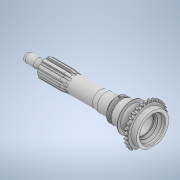
# Autodesk Inventor part: 68. Первичный вал
Saved by Autodesk Inventor 2021 (Build 250183000, 183)
## iProperties
Created: 2021-03-21
Part Number: 68. Первичный вал
Material: Типовые
Document SubType Name: Modeling
Designer: Данил
Density: 1 g/cm^3
Appearance: По умолчанию
Author: Данил
Autodesk Inventor part; units mm, degrees
sketch "Эскиз1" plane through (0, 0, 0) normal (0, 0, 1) x (1, 0, 0)
  line L0 (-123.25, 0) -> (123.25, 0)
  line L1 (-123.25, 0) -> (-123.25, -7.4282)
  line L2 (-119.25, -8.5) -> (-102.35, -8.5)
  line L3 (-119.25, -8.5) -> (-123.25, -7.4282)
  line L4 (-102.25, -8.6) -> (-102.25, -8.65)
  line L5 (-102.15, -8.75) -> (-91.25, -8.75)
  arc A0 (-102.25, -8.6) -> (-102.35, -8.5) centre (-102.35, -8.6) ccw
  arc A1 (-102.25, -8.65) -> (-102.15, -8.75) centre (-102.15, -8.65) ccw
  line L6 (-89.25, -10.75) -> (-89.25, -17.5)
  line L7 (-89.25, -17.5) -> (-43.25, -17.5)
  arc A2 (-89.25, -10.75) -> (-91.25, -8.75) centre (-91.25, -10.75) ccw
  line L8 (-43.25, -17.5) -> (-32.5769, -16)
  line L9 (-32.5769, -16) -> (20.5769, -16)
  line L10 (20.5769, -16) -> (31.25, -17.5)
  line L11 (31.25, -17.5) -> (50.5, -17.5)
  line L12 (50.5, -17.5) -> (50.6036, -17.3964)
  line L13 (50.9571, -17.25) -> (52.75, -17.25)
  line L14 (53.75, -18.25) -> (53.75, -21.5)
  arc A3 (50.9571, -17.25) -> (50.6036, -17.3964) centre (50.9571, -17.75) ccw
  arc A4 (53.75, -18.25) -> (52.75, -17.25) centre (52.75, -18.25) ccw
  line L15 (54.75, -22.5) -> (60.75, -22.5)
  line L16 (54.75, -22.5) -> (53.75, -21.5)
  line L17 (60.75, -22.5) -> (61.7036, -21.5464)
  line L18 (62.0571, -21.4) -> (63.35, -21.4)
  line L19 (64.35, -22.4) -> (64.35, -22.5)
  arc A5 (62.0571, -21.4) -> (61.7036, -21.5464) centre (62.0571, -21.9) ccw
  arc A6 (64.35, -22.4) -> (63.35, -21.4) centre (63.35, -22.4) ccw
  line L20 (64.35, -22.5) -> (78.1, -22.5)
  line L21 (78.1, -22.5) -> (78.2036, -22.3964)
  line L22 (78.5571, -22.25) -> (80.35, -22.25)
  line L23 (81.35, -23.25) -> (81.35, -28.25)
  arc A7 (78.5571, -22.25) -> (78.2036, -22.3964) centre (78.5571, -22.75) ccw
  arc A8 (81.35, -23.25) -> (80.35, -22.25) centre (80.35, -23.25) ccw
  line L24 (81.35, -28.25) -> (82.45, -28.25)
  line L25 (82.45, -28.25) -> (82.45, -36.4175)
  line L26 (82.45, -36.4175) -> (102.35, -36.4175)
  line L27 (102.35, -36.4175) -> (102.35, -30)
  line L28 (104.35, -28) -> (104.85, -28)
  line L29 (106.85, -30) -> (106.85, -40.5)
  arc A9 (104.35, -28) -> (102.35, -30) centre (104.35, -30) ccw
  arc A10 (106.85, -30) -> (104.85, -28) centre (104.85, -30) ccw
  line L30 (106.85, -40.5) -> (112.35, -40.5)
  line L31 (112.35, -40.5) -> (112.35, -32)
  line L32 (112.35, -32) -> (123.25, -31.5)
  line L33 (123.25, -31.5) -> (123.25, -26)
  line L34 (123.25, -26) -> (121.5179, -25)
  line L35 (121.5179, -25) -> (116.25, -25)
  line L36 (112.25, -21) -> (112.25, -20.4047)
  arc A11 (112.25, -21) -> (116.25, -25) centre (116.25, -21) ccw
  line L37 (112.25, -20.4047) -> (110.25, -19.25)
  line L38 (110.25, -19.25) -> (107.85, -19.25)
  line L39 (105.05, -19.25) -> (88.95, -19.25)
  line L40 (88.95, -19.25) -> (88.95, -19.75)
  line L41 (88.95, -19.75) -> (86.45, -19.75)
  line L42 (86.45, -19.75) -> (86.45, -15.6547)
  line L43 (86.45, -15.6547) -> (84.45, -14.5)
  line L44 (84.45, -14.5) -> (79.25, -14.5)
  line L45 (79.25, -14.5) -> (70.8784, 0)
  line L46 (105.05, -19.25) -> (105.05, -20.75)
  line L47 (106.05, -21.75) -> (106.85, -21.75)
  line L48 (107.85, -20.75) -> (107.85, -19.25)
  arc A12 (105.05, -20.75) -> (106.05, -21.75) centre (106.05, -20.75) ccw
  arc A13 (106.85, -21.75) -> (107.85, -20.75) centre (106.85, -20.75) ccw
  point P0 (0, 0)
  point P1 (0, 0)
  point P2 (-123.25, -8.5)
  point P3 (50.75, -17.25)
  point P4 (53.75, -22.5)
  point P5 (61.85, -21.4)
  point P6 (78.35, -22.25)
  point P7 (106.45, -21.75)
  dimension "d0" = 246.5
  dimension "d1" = 17
  dimension "d2" = 4
  dimension "d3" = 15
  dimension "d4" = 17.5
  dimension "d5" = 21
  dimension "d6" = 0.1
  dimension "d7" = 35
  dimension "d8" = 2
  dimension "d9" = 46
  dimension "d10" = 8
  dimension "d11" = 32
  dimension "d12" = 8
  dimension "d13" = 35
  dimension "d14" = 34
  dimension "d15" = 45
  dimension "d16" = 3
  dimension "d17" = 34.5
  dimension "d18" = 0.5
  dimension "d19" = 1
  dimension "d20" = 69.5
  dimension "d21" = 1
  dimension "d22" = 45
  dimension "d23" = 45
  dimension "d24" = 7
  dimension "d25" = 45
  dimension "d26" = 2.5
  dimension "d27" = 0.5
  dimension "d28" = 1
  dimension "d29" = 42.8
  dimension "d30" = 45
  dimension "d31" = 45
  dimension "d32" = 3
  dimension "d33" = 0.5
  dimension "d34" = 1
  dimension "d35" = 44.5
  dimension "d36" = 17
  dimension "d37" = 56.5
  dimension "d38" = 1.1
  dimension "d39" = 72.835
  dimension "d40" = 2
  dimension "d41" = 2
  dimension "d42" = 81
  dimension "d43" = 5.5
  dimension "d44" = 64
  dimension "d45" = 56
  dimension "d46" = 63
  dimension "d47" = 21
  dimension "d48" = 31
  dimension "d50" = 52
  dimension "d51" = 50
  dimension "d52" = 30
  dimension "d53" = 11
  dimension "d54" = 4
  dimension "d55" = 38.5
  dimension "d56" = 30
  dimension "d57" = 2
  dimension "d59" = 2.8
  dimension "d60" = 39.5
  dimension "d61" = 2.5
  dimension "d63" = 30
  dimension "d64" = 2
  dimension "d65" = 60
  dimension "d66" = 29
  constraints: 98 end point, 28 point on circle, 28 tangent, 15 horizontal, 14 centre point, 13 perpendicular, 11 point on line, 8 vertical, 2 coincident, 2 equal radius, 2 midpoint, 1 horizontal alignment, 1 vertical alignment
  measures "d0" distance of L0.start L0.end
  measures "d1" diameter of L2 L0
  measures "d2" distance of L2.start point (-123.25, -8.5)
  measures "d3" angle of L2 L3
  measures "d4" diameter of L5 L0
  measures "d5" distance from line of L0.start L4
  measures "d6" radius of A0
  measures "d7" diameter of L7 L0
  measures "d8" radius of A2
  measures "d9" distance from line of L7.end L6
  measures "d10" angle of L9 L8
  measures "d11" diameter of L9 L0
  measures "d12" angle of L11 L10
  measures "d13" diameter of L11 L0
  measures "d14" distance from line of L0.start L6
  measures "d15" angle of L14 L12
  measures "d16" distance from line of L14 point (50.75, -17.25)
  measures "d17" diameter of L13 L0
  measures "d18" radius of A3
  measures "d19" radius of A4
  measures "d20" distance from line of L0.end L14
  measures "d21" distance of L15.start point (53.75, -22.5)
  measures "d22" angle of L15 L16
  measures "d23" diameter of L15 L0
  measures "d24" distance from line of L15.end L14
  measures "d25" angle of L19 L17
  measures "d26" distance from line of L19 point (61.85, -21.4)
  measures "d27" radius of A5
  measures "d28" radius of A6
  measures "d29" diameter of L18 L0
  measures "d30" diameter of L20 L0
  measures "d31" angle of L21 L23
  measures "d32" distance from line of L23 point (78.35, -22.25)
  measures "d33" radius of A7
  measures "d34" radius of A8
  measures "d35" diameter of L22 L0
  measures "d36" distance between parallel lines of L23 L19
  measures "d37" diameter of L24 L0
  measures "d38" distance of L23.end L24.end
  measures "d39" diameter of L26 L0
  measures "d40" radius of A9
  measures "d41" radius of A10
  measures "d42" diameter of L30 L0
  measures "d43" distance of L29.end L30.end
  measures "d44" diameter of L31.end L0
  measures "d45" diameter of L28 L0
  measures "d46" diameter of L32.end L0
  measures "d47" distance between parallel lines of L27 L23
  measures "d48" distance between parallel lines of L31 L23
  measures "d50" diameter of L33.end L0
  measures "d51" diameter of L34.end L0
  measures "d52" angle of L35 L34
  measures "d53" distance between parallel lines of L36 L33
  measures "d54" radius of A11
  measures "d55" diameter of L38 L0
  measures "d56" angle of L38 L37
  measures "d57" horizontal distance of L36.end L37.end
  measures "d59" distance of L38.end L39.start
  measures "d60" diameter of L41 L0
  measures "d61" distance of L40.end L41.end
  measures "d63" angle of L39 L43
  measures "d64" distance from line of L43.end L42
  measures "d65" angle of L0 L45
  measures "d66" diameter of L44 L0
revolve "Вращение1" add sketch "Эскиз1" angle 360 about axis through (-123.25, 0, 0) along (1, 0, 0)
thread "Резьба1" size "M45x1.5" class "6g" standard "ISO Metric profile" full length
ref_plane "РабПлоскость1" through (104.6, 0, 0) normal (-1, 0, 0) x (0, 0, 1)
sketch "Эскиз2" plane through (104.6, 0, 0) normal (-1, 0, 0) x (0, 0, 1)
  line L0 (8, 36.4175) -> (-8, 36.4175) construction
  circle A0 centre (0, 0) radius 36.4175 projected
  line L1 (8, -35.5279) -> (8, 35.5279)
  line L2 (-8, 35.5279) -> (-8, -35.5279)
  line L3 (-8, 26.8328) -> (-9.5, 26.8328)
  line L4 (-9.5, 26.8328) -> (-9.5, 16.7425)
  line L5 (-9.5, 16.7425) -> (-8, 16.7425)
  circle A1 centre (0, 0) radius 28 projected
  circle A2 centre (0, 0) radius 19.25 projected
  line L6 (8, -16.6854) -> (9.6, -16.6854)
  line L7 (9.6, -16.6854) -> (9.6, -26.8328)
  line L8 (9.6, -26.8328) -> (8, -26.8328)
  point P0 (0, 36.4175)
  dimension "d74" = 16
  dimension "d75" = 3
  dimension "d76" = 3.2
  constraints: 18 end point, 8 point on circle, 4 horizontal, 4 point on line, 3 perpendicular, 3 vertical alignment, 2 vertical, 1 midpoint, 1 tangent
  measures "d74" distance of L0.start L0.end
  measures "d75" diameter of L4 L2
  measures "d76" diameter of L7 L1
revolve "Вращение2" cut sketch "Эскиз2" angle 360 about axis through (104.6, -35.5279, 8) along (0, 1, 0) picked at (8.7139, -20.3543) picked at (8.8918, -16.7824) contours L1 A2 L7 A1 | A1 L7 L8 | L1 L6 A2
revolve "Вращение3" cut sketch "Эскиз2" angle 360 about axis through (104.6, 35.5279, -8) along (0, -1, 0) picked at (-8.6691, 20.372) picked at (-8.8359, 16.8325) contours A1 L4 L3 | L2 A2 L4 A1 | L2 L5 A2
sketch "Эскиз3" plane through (0, 0, 0) normal (0, 0, 1) x (1, 0, 0)
  line L0 (50.5, 17.5) -> (31.25, 17.5) projected
  line L1 (70.8784, 0) -> (79.25, -14.5) projected
  line L2 (83.9986, -8.3348) -> (48.5273, 22.5)
  line L3 (70.8784, 0) -> (79.25, 14.5) projected
  line L4 (64.3813, 5.6018) -> (64.3663, 5.5844)
  line L5 (64.3311, 5.5818) -> (46.8871, 20.6132)
  line L6 (60.75, 22.5) -> (54.75, 22.5) projected
  line L7 (46.8871, 20.6132) -> (48.5273, 22.5)
  line L8 (78.1, -22.5) -> (64.35, -22.5) projected
  arc A0 (64.3311, 5.5818) -> (64.3663, 5.5844) centre (64.3474, 5.6007) ccw
  arc A1 (64.4166, 5.6044) -> (64.3813, 5.6018) centre (64.4003, 5.5855) ccw
  line L9 (83.9986, -8.3348) -> (82.4916, -10.0723)
  line L10 (64.4166, 5.6044) -> (82.4916, -10.0723)
  point P0 (0, 0)
  point P1 (64.35, 5.5655)
  point P2 (72.0587, 2.0444)
  point P3 (64.3659, 5.584)
  dimension "d79" = 41
  dimension "d81" = 4.8
  dimension "d82" = 5
  dimension "d83" = 0.025
  dimension "d89" = 4.6
  dimension "d90" = 47
  constraints: 12 end point, 4 point on circle, 4 point on line, 4 tangent, 3 perpendicular, 2 centre point, 1 equal radius, 1 horizontal alignment, 1 vertical alignment
  measures "d79" angle of L0 L2
  measures "d81" diameter of point (64.35, 5.565) L2
  measures "d82" diameter of L5.end L2
  measures "d83" radius of A0
  measures "d89" diameter of L9.end L2
  measures "d90" distance of L2.start L2.end
revolve "Вращение4" cut sketch "Эскиз3" angle 360 about axis through (83.9986, -8.3348, 0) along (-0.7547096, 0.656059, 0)
sketch "Эскиз4" plane through (0, 0, 0) normal (0, 0, 1) x (1, 0, 0)
  line L0 (60.75, 22.5) -> (54.75, 22.5) projected
  line L1 (53.75, 18.0823) -> (53.75, -18.25) projected
  line L2 (53.75, 18.0823) -> (53.75, 21.2451) projected
  arc A0 (53.75, 19.5) -> (60.75, 22.5) centre (41.5648, 57.5988) ccw
  line L3 (54.75, 22.5) -> (53.75, 21.5) projected
  line L4 (53.75, 21.5) -> (53.75, -21.5) projected
  point P0 (0, 0)
  dimension "d85" = 40
  dimension "d86" = 3
  constraints: 2 point on circle, 1 centre point, 1 point on line
  measures "d85" radius of A0
  measures "d86" vertical distance of L0.start A0.start
extrude "Выдавливание1" cut sketch "Эскиз4" along normal mid plane 3
sketch "Эскиз5" plane through (-89.25, 0, 0) normal (-1, 0, 0) x (0, 0, 1)
  circle A0 centre (0, 0) radius 17.5 projected
  circle A1 centre (0, 0) radius 13.25
  line L0 (-1.4483, 13.1706) -> (-2.7827, 17.2773)
  line L1 (-6.5698, 11.5065) -> (-7.9041, 15.6133)
  line L2 (-6.5698, 11.5065) -> (-1.4483, 13.1706) construction
  line L3 (-8.9132, 9.8039) -> (-12.4066, 12.342)
  line L4 (-12.0784, 5.4474) -> (-15.5718, 7.9855)
  line L5 (-12.0784, 5.4474) -> (-8.9132, 9.8039) construction
  line L6 (-12.9735, 2.6925) -> (-17.2916, 2.6925)
  line L7 (-12.9735, -2.6925) -> (-17.2916, -2.6925)
  line L8 (-12.9735, -2.6925) -> (-12.9735, 2.6925) construction
  line L9 (-12.0784, -5.4474) -> (-15.5718, -7.9855)
  line L10 (-8.9132, -9.8039) -> (-12.4066, -12.342)
  line L11 (-8.9132, -9.8039) -> (-12.0784, -5.4474) construction
  line L12 (-6.5698, -11.5065) -> (-7.9041, -15.6133)
  line L13 (-1.4483, -13.1706) -> (-2.7827, -17.2773)
  line L14 (-1.4483, -13.1706) -> (-6.5698, -11.5065) construction
  line L15 (1.4483, -13.1706) -> (2.7827, -17.2773)
  line L16 (6.5698, -11.5065) -> (7.9041, -15.6133)
  line L17 (6.5698, -11.5065) -> (1.4483, -13.1706) construction
  line L18 (8.9132, -9.8039) -> (12.4066, -12.342)
  line L19 (12.0784, -5.4474) -> (15.5718, -7.9855)
  line L20 (12.0784, -5.4474) -> (8.9132, -9.8039) construction
  line L21 (12.9735, -2.6925) -> (17.2916, -2.6925)
  line L22 (12.9735, 2.6925) -> (17.2916, 2.6925)
  line L23 (12.9735, 2.6925) -> (12.9735, -2.6925) construction
  line L24 (12.0784, 5.4474) -> (15.5718, 7.9855)
  line L25 (8.9132, 9.8039) -> (12.4066, 12.342)
  line L26 (8.9132, 9.8039) -> (12.0784, 5.4474) construction
  line L27 (6.5698, 11.5065) -> (7.9041, 15.6133)
  line L28 (1.4483, 13.1706) -> (2.7827, 17.2773)
  line L29 (1.4483, 13.1706) -> (6.5698, 11.5065) construction
  line L30 (-1.4483, 13.1706) -> (1.4483, 13.1706) construction
  point P0 (0, 13.1706)
  dimension "d92" = 26.5
  dimension "d93" = 5.385
  dimension "d94" = 90
  dimension "d97" = 360
  constraints: 62 end point, 4 point on circle, 1 centre point, 1 coincident, 1 midpoint, 1 parallel, 1 vertical alignment, 71 other
  measures "d92" diameter of A1
  measures "d93" distance between parallel lines of L1 L0
  measures "d94" angle of L1 L2
extrude "Выдавливание2" cut sketch "Эскиз5" against normal blind 46 contours L22 A1 L24 A0 | A0 L19 A1 L21 | L25 A1 L27 A0 | A0 L16 A1 L18 | L28 A1 L0 A0 | A0 L13 A1 L15 | L1 A1 L3 A0 | A0 L10 A1 L12 | L4 A1 L6 A0 | A0 L7 A1 L9
sketch "Эскиз6" plane through (-43.25, 0, 0) normal (-1, 0, 0) x (0, 0, 1)
  arc A0 (2.7827, 17.2773) -> (-2.7827, 17.2773) centre (0, 0) ccw projected
  line L0 (-1.4483, 13.1706) -> (-2.7827, 17.2773) projected
  arc A1 (1.4483, 13.1706) -> (-1.4483, 13.1706) centre (0, 0) ccw projected
  line L1 (2.7827, 17.2773) -> (1.4483, 13.1706) projected
ref_plane "РабПлоскость2" through (-28.25, 0, 0) normal (-1, 0, 0) x (0, 0, 1)
sketch "Эскиз7" plane through (-28.25, 0, 0) normal (-1, 0, 0) x (0, 0, 1)
  arc A0 (2.7827, 17.2773) -> (-2.7827, 17.2773) centre (0, 0) ccw projected
  line L0 (2.7827, 17.2773) -> (1.4483, 13.1706) projected
  arc A1 (1.4483, 13.1706) -> (-1.4483, 13.1706) centre (0, 0) ccw projected
  line L1 (-1.4483, 13.1706) -> (-2.7827, 17.2773) projected
  circle A2 centre (0, 0) radius 16 projected
  circle A3 centre (0, 0) radius 16 projected
  line L2 (-2.313, 15.8319) -> (-2.7827, 17.2773)
  line L3 (2.313, 15.8319) -> (2.7827, 17.2773)
  arc A4 (2.313, 15.8319) -> (-2.313, 15.8319) centre (0, 0) ccw
  arc A5 (2.7827, 17.2773) -> (-2.7827, 17.2773) centre (0, 0) ccw
  constraints: 4 end point, 4 point on circle, 2 centre point, 2 point on line, 1 coincident, 1 collinear, 5 other
loft "Лофт1" cut profiles "Эскиз7" section 1 edges at (-43.25, 17.5, 0) (-43.25, 15.224, -2.1155) (-43.25, 13.25, 0) (-43.25, 15.224, 2.1155) contours L0 A2 L1 A0
pattern_circular "Круговой массив1" count 10 over 360 about axis through (-6, 0, 0) along (-1, 0, 0) of "Лофт1"
sketch "Эскиз8" plane through (0, 0, 0) normal (0, 1, 0) x (-1, 0, 0)
  line L0 (89.25, 12.4066) -> (89.25, 15.5718) projected
  line L1 (89.25, 12) -> (86.0746, 17.5)
  line L2 (43.25, 17.5) -> (89.25, 17.5) projected
  line L3 (89.25, 17.2916) -> (89.25, 17.5) projected
  line L4 (89.25, 17.2916) -> (89.25, 12.9735) projected
  line L5 (89.25, 12.0784) -> (89.25, 12.9735) projected
  line L6 (89.25, 12.4066) -> (89.25, 8.9132) projected
  line L7 (123.25, 0) -> (0, 0)
  line L8 (123.25, -7.4282) -> (123.25, 7.4282) projected
  dimension "d111" = 24
  dimension "d113" = 30
  constraints: 4 end point, 2 point on line, 1 horizontal, 1 midpoint
  measures "d111" diameter of L1.start L7
  measures "d113" angle of L4 L1
revolve "Вращение5" cut sketch "Эскиз8" angle 360 about axis through (-123.25, 0, 0) along (1, 0, 0)
sketch "Эскиз9" plane through (112.35, 0, 0) normal (1, 0, 0) x (0, 0, -1)
  circle A0 centre (0, 0) radius 40.5 projected
  circle A1 centre (0, 0) radius 32 projected
  circle A2 centre (0, 0) radius 39 construction
  circle A3 centre (0, 0) radius 40.5 projected
  circle A4 centre (0, 0) radius 37
  arc A5 (-1.4336, 40.4746) -> (-2.042, 36.9436) centre (5.9458, 37.3851) ccw
  arc A6 (2.042, 36.9436) -> (1.4336, 40.4746) centre (-5.9458, 37.3851) ccw
  line L0 (-2.042, 36.9436) -> (2.042, 36.9436) construction
  line L1 (-1.4336, 40.4746) -> (1.4336, 40.4746) construction
  arc A7 (-9.8174, 39.2921) -> (-9.6784, 35.7117) centre (-1.9569, 37.8044) ccw
  arc A8 (-5.6836, 36.5609) -> (-7.0129, 39.8882) centre (-13.5887, 35.332) ccw
  arc A9 (-17.7721, 36.3923) -> (-16.8918, 32.9191) centre (-9.7741, 36.5714) ccw
  arc A10 (-13.1609, 34.5802) -> (-15.1529, 37.5585) centre (-20.6377, 31.7346) ccw
  arc A11 (-24.9502, 31.902) -> (-23.3669, 28.6877) centre (-17.1642, 33.7401) ccw
  arc A12 (-20.0629, 31.0883) -> (-22.6306, 33.5873) centre (-26.7847, 26.7503) ccw
  arc A13 (-31.0377, 26.0175) -> (-28.8208, 23.2026) centre (-23.804, 29.4341) ccw
  arc A14 (-26.0881, 26.2376) -> (-29.1193, 28.1481) centre (-31.7611, 20.5969) ccw
  arc A15 (-35.7688, 18.9958) -> (-33.0151, 16.7034) centre (-29.4036, 23.8418) ccw
  arc A16 (-30.9731, 20.2402) -> (-34.3353, 21.4788) centre (-35.3494, 13.5433) ccw
  arc A17 (-38.9366, 11.144) -> (-35.7665, 9.4741) centre (-33.718, 17.2074) ccw
  arc A18 (-34.5044, 13.3583) -> (-38.0507, 13.8707) centre (-37.3927, 5.8978) ccw
  arc A19 (-40.4027, 2.805) -> (-36.9547, 1.8308) centre (-36.5588, 9.821) ccw
  arc A20 (-36.5278, 5.8925) -> (-40.103, 5.6565) centre (-37.8018, -2.0054) ccw
  arc A21 (-40.103, -5.6565) -> (-36.5278, -5.8925) centre (-37.8018, 2.0054) ccw
  arc A22 (-36.9547, -1.8308) -> (-40.4027, -2.805) centre (-36.5588, -9.821) ccw
  arc A23 (-38.0507, -13.8707) -> (-34.5044, -13.3583) centre (-37.3927, -5.8978) ccw
  arc A24 (-35.7665, -9.4741) -> (-38.9366, -11.144) centre (-33.718, -17.2074) ccw
  arc A25 (-34.3353, -21.4788) -> (-30.9731, -20.2402) centre (-35.3494, -13.5433) ccw
  arc A26 (-33.0151, -16.7034) -> (-35.7688, -18.9958) centre (-29.4036, -23.8418) ccw
  arc A27 (-29.1193, -28.1481) -> (-26.0881, -26.2376) centre (-31.7611, -20.5969) ccw
  arc A28 (-28.8208, -23.2026) -> (-31.0377, -26.0175) centre (-23.804, -29.4341) ccw
  arc A29 (-22.6306, -33.5873) -> (-20.0629, -31.0883) centre (-26.7847, -26.7503) ccw
  arc A30 (-23.3669, -28.6877) -> (-24.9502, -31.902) centre (-17.1642, -33.7401) ccw
  arc A31 (-15.1529, -37.5585) -> (-13.1609, -34.5802) centre (-20.6377, -31.7346) ccw
  arc A32 (-16.8918, -32.9191) -> (-17.7721, -36.3923) centre (-9.7741, -36.5714) ccw
  arc A33 (-7.0129, -39.8882) -> (-5.6836, -36.5609) centre (-13.5887, -35.332) ccw
  arc A34 (-9.6784, -35.7117) -> (-9.8174, -39.2921) centre (-1.9569, -37.8044) ccw
  arc A35 (1.4336, -40.4746) -> (2.042, -36.9436) centre (-5.9458, -37.3851) ccw
  arc A36 (-2.042, -36.9436) -> (-1.4336, -40.4746) centre (5.9458, -37.3851) ccw
  arc A37 (9.8174, -39.2921) -> (9.6784, -35.7117) centre (1.9569, -37.8044) ccw
  arc A38 (5.6836, -36.5609) -> (7.0129, -39.8882) centre (13.5887, -35.332) ccw
  arc A39 (17.7721, -36.3923) -> (16.8918, -32.9191) centre (9.7741, -36.5714) ccw
  arc A40 (13.1609, -34.5802) -> (15.1529, -37.5585) centre (20.6377, -31.7346) ccw
  arc A41 (24.9502, -31.902) -> (23.3669, -28.6877) centre (17.1642, -33.7401) ccw
  arc A42 (20.0629, -31.0883) -> (22.6306, -33.5873) centre (26.7847, -26.7503) ccw
  arc A43 (31.0377, -26.0175) -> (28.8208, -23.2026) centre (23.804, -29.4341) ccw
  arc A44 (26.0881, -26.2376) -> (29.1193, -28.1481) centre (31.7611, -20.5969) ccw
  arc A45 (35.7688, -18.9958) -> (33.0151, -16.7034) centre (29.4036, -23.8418) ccw
  arc A46 (30.9731, -20.2402) -> (34.3353, -21.4788) centre (35.3494, -13.5433) ccw
  arc A47 (38.9366, -11.144) -> (35.7665, -9.4741) centre (33.718, -17.2074) ccw
  arc A48 (34.5044, -13.3583) -> (38.0507, -13.8707) centre (37.3927, -5.8978) ccw
  arc A49 (40.4027, -2.805) -> (36.9547, -1.8308) centre (36.5588, -9.821) ccw
  arc A50 (36.5278, -5.8925) -> (40.103, -5.6565) centre (37.8018, 2.0054) ccw
  arc A51 (40.103, 5.6565) -> (36.5278, 5.8925) centre (37.8018, -2.0054) ccw
  arc A52 (36.9547, 1.8308) -> (40.4027, 2.805) centre (36.5588, 9.821) ccw
  arc A53 (38.0507, 13.8707) -> (34.5044, 13.3583) centre (37.3927, 5.8978) ccw
  arc A54 (35.7665, 9.4741) -> (38.9366, 11.144) centre (33.718, 17.2074) ccw
  arc A55 (34.3353, 21.4788) -> (30.9731, 20.2402) centre (35.3494, 13.5433) ccw
  arc A56 (33.0151, 16.7034) -> (35.7688, 18.9958) centre (29.4036, 23.8418) ccw
  arc A57 (29.1193, 28.1481) -> (26.0881, 26.2376) centre (31.7611, 20.5969) ccw
  arc A58 (28.8208, 23.2026) -> (31.0377, 26.0175) centre (23.804, 29.4341) ccw
  arc A59 (22.6306, 33.5873) -> (20.0629, 31.0883) centre (26.7847, 26.7503) ccw
  arc A60 (23.3669, 28.6877) -> (24.9502, 31.902) centre (17.1642, 33.7401) ccw
  arc A61 (15.1529, 37.5585) -> (13.1609, 34.5802) centre (20.6377, 31.7346) ccw
  arc A62 (16.8918, 32.9191) -> (17.7721, 36.3923) centre (9.7741, 36.5714) ccw
  arc A63 (7.0129, 39.8882) -> (5.6836, 36.5609) centre (13.5887, 35.332) ccw
  arc A64 (9.6784, 35.7117) -> (9.8174, 39.2921) centre (1.9569, 37.8044) ccw
  point P0 (0, 37)
  point P1 (0, 40.5)
  point P2 (0, 36.9436)
  point P3 (0, 40.4746)
  point P4 (-15.1529, 37.5585)
  point P5 (-9.6784, 35.7117)
  point P6 (-9.8174, 39.2921)
  point P7 (-20.0629, 31.0883)
  point P8 (-16.8918, 32.9191)
  point P9 (-17.7721, 36.3923)
  point P10 (-23.3669, 28.6877)
  point P11 (-24.9502, 31.902)
  point P12 (-30.9731, 20.2402)
  point P13 (-28.8208, 23.2026)
  point P14 (-31.0377, 26.0175)
  point P15 (-34.5044, 13.3583)
  point P16 (-33.0151, 16.7034)
  point P17 (-35.7688, 18.9958)
  point P18 (-40.103, 5.6565)
  point P19 (-35.7665, 9.4741)
  point P20 (-38.9366, 11.144)
  point P21 (-40.4027, -2.805)
  point P22 (-36.9547, -1.8308)
  point P23 (-36.9547, 1.8308)
  point P24 (-40.4027, 2.805)
  point P25 (-38.9366, -11.144)
  point P26 (-35.7665, -9.4741)
  point P27 (-36.5278, -5.8925)
  point P28 (-40.103, -5.6565)
  point P29 (-35.7688, -18.9958)
  point P30 (-34.5044, -13.3583)
  point P31 (-38.0507, -13.8707)
  point P32 (-30.9731, -20.2402)
  point P33 (-34.3353, -21.4788)
  point P34 (-24.9502, -31.902)
  point P35 (-26.0881, -26.2376)
  point P36 (-29.1193, -28.1481)
  point P37 (-17.7721, -36.3923)
  point P38 (-16.8918, -32.9191)
  point P39 (-20.0629, -31.0883)
  point P40 (-22.6306, -33.5873)
  point P41 (-9.8174, -39.2921)
  point P42 (-9.6784, -35.7117)
  point P43 (-13.1609, -34.5802)
  point P44 (-15.1529, -37.5585)
  point P45 (-1.4336, -40.4746)
  point P46 (-2.042, -36.9436)
  point P47 (-5.6836, -36.5609)
  point P48 (-7.0129, -39.8882)
  point P49 (7.0129, -39.8882)
  point P50 (5.6836, -36.5609)
  point P51 (2.042, -36.9436)
  point P52 (1.4336, -40.4746)
  point P53 (15.1529, -37.5585)
  point P54 (13.1609, -34.5802)
  point P55 (9.6784, -35.7117)
  point P56 (9.8174, -39.2921)
  point P57 (22.6306, -33.5873)
  point P58 (20.0629, -31.0883)
  point P59 (16.8918, -32.9191)
  point P60 (17.7721, -36.3923)
  point P61 (29.1193, -28.1481)
  point P62 (23.3669, -28.6877)
  point P63 (24.9502, -31.902)
  point P64 (28.8208, -23.2026)
  point P65 (31.0377, -26.0175)
  point P66 (34.5044, -13.3583)
  point P67 (33.0151, -16.7034)
  point P68 (35.7688, -18.9958)
  point P69 (40.103, -5.6565)
  point P70 (36.5278, -5.8925)
  point P71 (35.7665, -9.4741)
  point P72 (38.9366, -11.144)
  point P73 (40.4027, 2.805)
  point P74 (36.9547, 1.8308)
  point P75 (36.9547, -1.8308)
  point P76 (40.4027, -2.805)
  point P77 (38.9366, 11.144)
  point P78 (36.5278, 5.8925)
  point P79 (40.103, 5.6565)
  point P80 (34.5044, 13.3583)
  point P81 (38.0507, 13.8707)
  point P82 (31.0377, 26.0175)
  point P83 (28.8208, 23.2026)
  point P84 (30.9731, 20.2402)
  point P85 (34.3353, 21.4788)
  point P86 (24.9502, 31.902)
  point P87 (26.0881, 26.2376)
  point P88 (29.1193, 28.1481)
  point P89 (17.7721, 36.3923)
  point P90 (16.8918, 32.9191)
  point P91 (20.0629, 31.0883)
  point P92 (22.6306, 33.5873)
  point P93 (9.8174, 39.2921)
  point P94 (9.6784, 35.7117)
  point P95 (13.1609, 34.5802)
  point P96 (15.1529, 37.5585)
  point P97 (5.6836, 36.5609)
  point P98 (7.0129, 39.8882)
  point P99 (1.4336, 40.4746)
  point P100 (-7.0129, 39.8882)
  point P101 (-5.6836, 36.5609)
  point P102 (-1.4336, 40.4746)
  dimension "d114" = 78
  dimension "d115" = 3.5
  dimension "d116" = 4.084
  dimension "d117" = 8
  dimension "d120" = 360
  constraints: 123 point on circle, 61 centre point, 4 end point, 4 vertical alignment, 2 coincident, 2 midpoint, 1 horizontal, 249 other
  measures "d114" diameter of A2
  measures "d115" distance of point (0, 37) A3.start
  measures "d116" distance of L0.start L0.end
  measures "d117" radius of A6
extrude "Выдавливание3" cut sketch "Эскиз9" against normal up to surface (5.5 mm away) contours A0 A49 A4 A52 | A51 A4 A54 A0 | A0 A47 A4 A50 | A53 A4 A56 A0 | A0 A45 A4 A48 | A55 A4 A58 A0 | A0 A43 A4 A46 | A57 A4 A60 A0 | A0 A41 A4 A44 | A59 A4 A62 A0 | A0 A39 A4 A42 | A61 A4 A64 A0 | A0 A37 A4 A40 | A63 A4 A6 A0 | A0 A35 A4 A38 | A5 A4 A8 A0 | A0 A33 A4 A36 | A7 A4 A10 A0 | A0 A31 A4 A34 | A9 A4 A12 A0 | A0 A29 A4 A32 | A11 A4 A14 A0 | A0 A27 A4 A30 | A13 A4 A16 A0 | A0 A25 A4 A28 | A15 A4 A18 A0 | A0 A23 A4 A26 | A17 A4 A20 A0 | A0 A21 A4 A24 | A19 A4 A22 A0
ref_plane "РабПлоскость3" through (0, 40.5, 0) normal (0, 1, 0) x (-1, 0, 0)
sketch "Эскиз10" plane through (0, 40.5, 0) normal (0, 1, 0) x (-1, 0, 0)
  line L0 (-112.35, -1.4336) -> (-112.35, 1.4336) projected
  line L1 (-112.35, 2.0542) -> (-112.35, 1.4336) projected
  line L2 (-112.35, -1.4336) -> (-112.35, -2.0542) projected
  line L3 (-112.35, -1.4336) -> (-106.85, -1.4336) projected
  line L4 (-106.85, 1.4336) -> (-112.35, 1.4336) projected
  line L5 (-112.35, -0.25) -> (-110.6235, -2.5)
  line L6 (-112.35, 0.25) -> (-110.6235, 2.5)
  line L7 (-112.35, 0.25) -> (-112.35, -0.25) construction
  line L8 (-112.35, 5.6836) -> (-112.35, 2.042) projected
  line L9 (-112.35, -2.042) -> (-112.35, -5.6836) projected
  line L10 (-110.6235, 2.5) -> (-112.35, 2.5)
  line L11 (-110.6235, -2.5) -> (-112.35, -2.5)
  line L12 (-110.6235, 2.5) -> (-110.6235, -2.5) construction
  line L13 (-112.35, 2.042) -> (-106.85, 2.042) projected
  point P0 (0, 0)
  point P1 (-112.35, 0)
  point P2 (-110.6235, 0)
  dimension "d125" = 0.5
  dimension "d126" = 105
  dimension "d127" = 5
  constraints: 12 end point, 4 point on line, 2 horizontal alignment, 2 midpoint, 2 perpendicular, 1 collinear, 1 horizontal, 1 vertical alignment
  measures "d125" distance of L6.start L5.start
  measures "d126" angle of L6 L5
  measures "d127" distance between parallel lines of L10 L11
extrude "Выдавливание4" cut sketch "Эскиз10" against normal up to surface round surface about axis through (112.35, 0, 0) along (-1, 0, 0) radius 37 far side no
pattern_circular "Круговой массив2" count 30 over 360 about axis through (92.4, 0, 0) along (-1, 0, 0) of "Выдавливание4"
sketch "Эскиз11" plane through (112.35, 0, 0) normal (1, 0, 0) x (0, 0, -1)
  circle A0 centre (0, 0) radius 32 projected
  line L0 (-8.6648, 39.5622) -> (-7.9371, 36.1387) projected
  arc A1 (-7.9371, 36.1387) -> (-14.8205, 33.9021) centre (0, 0) ccw projected
  line L1 (-14.8205, 33.9021) -> (-16.2441, 37.0996) projected
  arc A2 (-16.2441, 37.0996) -> (-16.7009, 36.8962) centre (0, 0) ccw projected
  line L2 (-16.7009, 36.8962) -> (-15.2773, 33.6987) projected
  arc A3 (-15.2773, 33.6987) -> (-21.5453, 30.0799) centre (0, 0) ccw projected
  line L3 (-21.5453, 30.0799) -> (-23.6026, 32.9115) projected
  arc A4 (-23.6026, 32.9115) -> (-24.0071, 32.6176) centre (0, 0) ccw projected
  line L4 (-24.0071, 32.6176) -> (-21.9498, 29.786) projected
  arc A5 (-21.9498, 29.786) -> (-27.3284, 24.9431) centre (0, 0) ccw projected
  line L5 (-27.3284, 24.9431) -> (-29.9295, 27.2851) projected
  arc A6 (-29.9295, 27.2851) -> (-30.2641, 26.9135) centre (0, 0) ccw projected
  line L6 (-30.2641, 26.9135) -> (-27.663, 24.5715) projected
  arc A7 (-27.663, 24.5715) -> (-31.9172, 18.7161) centre (0, 0) ccw projected
  line L7 (-31.9172, 18.7161) -> (-34.9484, 20.4661) projected
  arc A8 (-34.9484, 20.4661) -> (-35.1984, 20.0331) centre (0, 0) ccw projected
  line L8 (-35.1984, 20.0331) -> (-32.1672, 18.2831) projected
  arc A9 (-32.1672, 18.2831) -> (-35.111, 11.6711) centre (0, 0) ccw projected
  line L9 (-35.111, 11.6711) -> (-38.4398, 12.7527) projected
  arc A10 (-38.4398, 12.7527) -> (-38.5943, 12.2772) centre (0, 0) ccw projected
  line L10 (-38.5943, 12.2772) -> (-35.2655, 11.1956) projected
  arc A11 (-35.2655, 11.1956) -> (-36.7703, 4.1161) centre (0, 0) ccw projected
  line L11 (-36.7703, 4.1161) -> (-40.2512, 4.482) projected
  arc A12 (-40.2512, 4.482) -> (-40.3035, 3.9847) centre (0, 0) ccw projected
  line L12 (-40.3035, 3.9847) -> (-36.8226, 3.6188) projected
  arc A13 (-36.8226, 3.6188) -> (-36.8226, -3.6188) centre (0, 0) ccw projected
  line L13 (-36.8226, -3.6188) -> (-40.3035, -3.9847) projected
  arc A14 (-40.3035, -3.9847) -> (-40.2512, -4.482) centre (0, 0) ccw projected
  line L14 (-40.2512, -4.482) -> (-36.7703, -4.1161) projected
  arc A15 (-36.7703, -4.1161) -> (-35.2655, -11.1956) centre (0, 0) ccw projected
  line L15 (-35.2655, -11.1956) -> (-38.5943, -12.2772) projected
  arc A16 (-38.5943, -12.2772) -> (-38.4398, -12.7527) centre (0, 0) ccw projected
  line L16 (-38.4398, -12.7527) -> (-35.111, -11.6711) projected
  arc A17 (-35.111, -11.6711) -> (-32.1672, -18.2831) centre (0, 0) ccw projected
  line L17 (-32.1672, -18.2831) -> (-35.1984, -20.0331) projected
  arc A18 (-35.1984, -20.0331) -> (-34.9484, -20.4661) centre (0, 0) ccw projected
  line L18 (-34.9484, -20.4661) -> (-31.9172, -18.7161) projected
  arc A19 (-31.9172, -18.7161) -> (-27.663, -24.5715) centre (0, 0) ccw projected
  line L19 (-27.663, -24.5715) -> (-30.2641, -26.9135) projected
  arc A20 (-30.2641, -26.9135) -> (-29.9295, -27.2851) centre (0, 0) ccw projected
  line L20 (-29.9295, -27.2851) -> (-27.3284, -24.9431) projected
  arc A21 (-27.3284, -24.9431) -> (-21.9498, -29.786) centre (0, 0) ccw projected
  line L21 (-21.9498, -29.786) -> (-24.0071, -32.6176) projected
  arc A22 (-24.0071, -32.6176) -> (-23.6026, -32.9115) centre (0, 0) ccw projected
  line L22 (-23.6026, -32.9115) -> (-21.5453, -30.0799) projected
  arc A23 (-21.5453, -30.0799) -> (-15.2773, -33.6987) centre (0, 0) ccw projected
  line L23 (-15.2773, -33.6987) -> (-16.7009, -36.8962) projected
  arc A24 (-16.7009, -36.8962) -> (-16.2441, -37.0996) centre (0, 0) ccw projected
  line L24 (-16.2441, -37.0996) -> (-14.8205, -33.9021) projected
  arc A25 (-14.8205, -33.9021) -> (-7.9371, -36.1387) centre (0, 0) ccw projected
  line L25 (-7.9371, -36.1387) -> (-8.6648, -39.5622) projected
  arc A26 (-8.6648, -39.5622) -> (-8.1757, -39.6662) centre (0, 0) ccw projected
  line L26 (-8.1757, -39.6662) -> (-7.448, -36.2426) projected
  arc A27 (-7.448, -36.2426) -> (-0.25, -36.9992) centre (0, 0) ccw projected
  line L27 (-0.25, -36.9992) -> (-0.25, -40.4992) projected
  arc A28 (-0.25, -40.4992) -> (0.25, -40.4992) centre (0, 0) ccw projected
  line L28 (0.25, -40.4992) -> (0.25, -36.9992) projected
  arc A29 (0.25, -36.9992) -> (7.448, -36.2426) centre (0, 0) ccw projected
  line L29 (7.448, -36.2426) -> (8.1757, -39.6662) projected
  arc A30 (8.1757, -39.6662) -> (8.6648, -39.5622) centre (0, 0) ccw projected
  line L30 (8.6648, -39.5622) -> (7.9371, -36.1387) projected
  arc A31 (7.9371, -36.1387) -> (14.8205, -33.9021) centre (0, 0) ccw projected
  line L31 (14.8205, -33.9021) -> (16.2441, -37.0996) projected
  arc A32 (16.2441, -37.0996) -> (16.7009, -36.8962) centre (0, 0) ccw projected
  line L32 (16.7009, -36.8962) -> (15.2773, -33.6987) projected
  arc A33 (15.2773, -33.6987) -> (21.5453, -30.0799) centre (0, 0) ccw projected
  line L33 (21.5453, -30.0799) -> (23.6026, -32.9115) projected
  arc A34 (23.6026, -32.9115) -> (24.0071, -32.6176) centre (0, 0) ccw projected
  line L34 (24.0071, -32.6176) -> (21.9498, -29.786) projected
  arc A35 (21.9498, -29.786) -> (27.3284, -24.9431) centre (0, 0) ccw projected
  line L35 (27.3284, -24.9431) -> (29.9295, -27.2851) projected
  arc A36 (29.9295, -27.2851) -> (30.2641, -26.9135) centre (0, 0) ccw projected
  line L36 (30.2641, -26.9135) -> (27.663, -24.5715) projected
  arc A37 (27.663, -24.5715) -> (31.9172, -18.7161) centre (0, 0) ccw projected
  line L37 (31.9172, -18.7161) -> (34.9484, -20.4661) projected
  arc A38 (34.9484, -20.4661) -> (35.1984, -20.0331) centre (0, 0) ccw projected
  line L38 (35.1984, -20.0331) -> (32.1672, -18.2831) projected
  arc A39 (32.1672, -18.2831) -> (35.111, -11.6711) centre (0, 0) ccw projected
  line L39 (35.111, -11.6711) -> (38.4398, -12.7527) projected
  arc A40 (38.4398, -12.7527) -> (38.5943, -12.2772) centre (0, 0) ccw projected
  line L40 (38.5943, -12.2772) -> (35.2655, -11.1956) projected
  arc A41 (35.2655, -11.1956) -> (36.7703, -4.1161) centre (0, 0) ccw projected
  line L41 (36.7703, -4.1161) -> (40.2512, -4.482) projected
  arc A42 (40.2512, -4.482) -> (40.3035, -3.9847) centre (0, 0) ccw projected
  line L42 (40.3035, -3.9847) -> (36.8226, -3.6188) projected
  arc A43 (36.8226, -3.6188) -> (36.8226, 3.6188) centre (0, 0) ccw projected
  line L43 (36.8226, 3.6188) -> (40.3035, 3.9847) projected
  arc A44 (40.3035, 3.9847) -> (40.2512, 4.482) centre (0, 0) ccw projected
  line L44 (40.2512, 4.482) -> (36.7703, 4.1161) projected
  arc A45 (36.7703, 4.1161) -> (35.2655, 11.1956) centre (0, 0) ccw projected
  line L45 (35.2655, 11.1956) -> (38.5943, 12.2772) projected
  arc A46 (38.5943, 12.2772) -> (38.4398, 12.7527) centre (0, 0) ccw projected
  line L46 (38.4398, 12.7527) -> (35.111, 11.6711) projected
  arc A47 (35.111, 11.6711) -> (32.1672, 18.2831) centre (0, 0) ccw projected
  line L47 (32.1672, 18.2831) -> (35.1984, 20.0331) projected
  arc A48 (35.1984, 20.0331) -> (34.9484, 20.4661) centre (0, 0) ccw projected
  line L48 (34.9484, 20.4661) -> (31.9172, 18.7161) projected
  arc A49 (31.9172, 18.7161) -> (27.663, 24.5715) centre (0, 0) ccw projected
  line L49 (27.663, 24.5715) -> (30.2641, 26.9135) projected
  arc A50 (30.2641, 26.9135) -> (29.9295, 27.2851) centre (0, 0) ccw projected
  line L50 (29.9295, 27.2851) -> (27.3284, 24.9431) projected
  arc A51 (27.3284, 24.9431) -> (21.9498, 29.786) centre (0, 0) ccw projected
  line L51 (21.9498, 29.786) -> (24.0071, 32.6176) projected
  arc A52 (24.0071, 32.6176) -> (23.6026, 32.9115) centre (0, 0) ccw projected
  line L52 (23.6026, 32.9115) -> (21.5453, 30.0799) projected
  arc A53 (21.5453, 30.0799) -> (15.2773, 33.6987) centre (0, 0) ccw projected
  line L53 (15.2773, 33.6987) -> (16.7009, 36.8962) projected
  arc A54 (16.7009, 36.8962) -> (16.2441, 37.0996) centre (0, 0) ccw projected
  line L54 (16.2441, 37.0996) -> (14.8205, 33.9021) projected
  arc A55 (14.8205, 33.9021) -> (7.9371, 36.1387) centre (0, 0) ccw projected
  line L55 (7.9371, 36.1387) -> (8.6648, 39.5622) projected
  arc A56 (8.6648, 39.5622) -> (8.1757, 39.6662) centre (0, 0) ccw projected
  line L56 (8.1757, 39.6662) -> (7.448, 36.2426) projected
  arc A57 (7.448, 36.2426) -> (0.25, 36.9992) centre (0, 0) ccw projected
  line L57 (0.25, 36.9992) -> (0.25, 40.4992) projected
  arc A58 (0.25, 40.4992) -> (-0.25, 40.4992) centre (0, 0) ccw projected
  line L58 (-0.25, 40.4992) -> (-0.25, 36.9992) projected
  arc A59 (-0.25, 36.9992) -> (-7.448, 36.2426) centre (0, 0) ccw projected
  line L59 (-7.448, 36.2426) -> (-8.1757, 39.6662) projected
  arc A60 (-8.1757, 39.6662) -> (-8.6648, 39.5622) centre (0, 0) ccw projected
  arc A61 (114.0132, -50) -> (-114.0132, -50) centre (0, -349) ccw
  arc A62 (1.4336, 40.4746) -> (-1.4336, 40.4746) centre (0, 0) ccw projected
  line L60 (-114.0132, -50) -> (114.0132, -50)
  point P0 (0, -29)
  point P1 (0, 40.5)
  point P2 (12.9509, -29.2622)
  point P3 (-12.9509, -29.2622)
  dimension "d133" = 320
  dimension "d134" = 69.5
  dimension "d135" = 50
  constraints: 5 point on circle, 2 end point, 2 vertical alignment, 1 centre point, 1 horizontal
  measures "d133" radius of A61
  measures "d134" distance of point (0, -29) point (0, 40.5)
  measures "d135" distance from line of point (0, 0) L60
extrude "Выдавливание5" cut sketch "Эскиз11" along normal blind 18.75 and the other way blind 7.875 contours A61 A0 | A0 A61 A35 L34 A34 L33 A33 L32 A32 L31 A31 L30 A30 L29 A29 L28 A28 L27 A27 L26 A26 L25 A25 L24 A24 L23 A23 L22 A22 L21 A21 | A21 L21 A22 L22 A23 L23 A24 L24 A25 L25 A26 L26 A27 L27 A28 L28 A29 L29 A30 L30 A31 L31 A32 L32 A33 L33 A34 L34 A35 A61 L60 picked at (0, -30.0194)
sketch "Эскиз12" plane through (112.35, 0, 0) normal (1, 0, 0) x (0, 0, -1)
  arc A0 (-26.0881, -26.2376) -> (-23.3669, -28.6877) centre (0, 0) ccw projected
  arc A1 (23.3669, -28.6877) -> (26.0881, -26.2376) centre (0, 0) ccw projected
  arc A2 (-25, -27.2764) -> (25, -27.2764) centre (0, 0) ccw
  circle A3 centre (0, 0) radius 17.5 projected
  arc A4 (-27.027, -29.488) -> (27.027, -29.488) centre (0, 0) ccw
  line L0 (-25, -27.2764) -> (-27.027, -29.488)
  line L1 (25, -27.2764) -> (27.027, -29.488)
  line L2 (-25, -27.2764) -> (25, -27.2764) construction
  point P0 (0, -27.2764)
  point P1 (23.3669, -28.6877)
  point P2 (-23.3669, -28.6877)
  dimension "d140" = 40
  dimension "d141" = 50
  constraints: 6 end point, 6 point on circle, 2 centre point, 2 coincident, 2 line through centre, 1 horizontal, 1 midpoint, 1 vertical alignment
  measures "d140" radius of A4
  measures "d141" distance of L0.start L1.start
extrude "Выдавливание6" cut sketch "Эскиз12" against normal up to surface (10 mm away) contours A0 A2 A1 L1 A4 L0
sketch "Эскиз13" plane through (112.35, 0, 0) normal (1, 0, 0) x (0, 0, -1)
  arc A0 (-36.7703, -4.1161) -> (-35.2655, -11.1956) centre (0, 0) ccw projected
  arc A1 (-36.2952, -7.5218) -> (-36.2167, -7.8911) centre (-36.1915, -7.6927) ccw
  arc A2 (-40.103, -5.6565) -> (-36.5278, -5.8925) centre (-37.8018, 2.0054) ccw projected
  arc A3 (-36.5278, -5.8925) -> (-36.2491, -7.4162) centre (0, 0) ccw
  arc A4 (-36.2952, -7.5218) -> (-36.2491, -7.4162) centre (-36.3471, -7.4363) ccw
  arc A5 (-35.7665, -9.4741) -> (-38.9366, -11.144) centre (-33.718, -17.2074) ccw projected
  arc A6 (-36.1317, -7.9688) -> (-35.7665, -9.4741) centre (0, 0) ccw
  arc A7 (-36.1317, -7.9688) -> (-36.2167, -7.8911) centre (-36.2293, -7.9903) ccw
  point P0 (-36.1915, -7.6927)
  point P1 (-36.1317, -7.9688)
  point P2 (-36.2491, -7.4162)
  dimension "d144" = 0.2
  dimension "d146" = 0.1
  dimension "d147" = 0.1
  constraints: 11 point on circle, 6 tangent, 5 centre point, 2 concentric, 1 coincident
  measures "d146" radius of A4
  measures "d147" radius of A7
extrude "Выдавливание7" add sketch "Эскиз13" against normal up to surface (5.5 mm away)
pattern_circular "Круговой массив3" count 4 over 36 about axis through (117.8, 0, 0) along (-1, 0, 0) of "Выдавливание7"
pattern_circular "Круговой массив4" count 2 over 360 about axis through (117.8, 0, 0) along (-1, 0, 0) of "Выдавливание7", "Круговой массив3"
sketch "Эскиз14" plane through (0, 0, 0) normal (0, 0, 1) x (1, 0, 0)
  line L0 (82.45, 36.4175) -> (82.45, -36.4175) projected
  line L1 (102.35, 30) -> (102.35, -30) projected
  line L2 (82.45, 36.4175) -> (102.35, 36.4175)
  line L3 (102.35, 36.4175) -> (102.35, 22.5)
  line L4 (102.35, 22.5) -> (82.45, 22.5)
  line L5 (82.45, 22.5) -> (82.45, 36.4175)
  line L6 (82.45, 28.25) -> (82.45, -28.25) projected
  line L7 (82.45, 0) -> (102.35, 0)
  point P0 (0, 0)
  point P1 (102.35, 30)
  dimension "d156" = 45
  constraints: 10 end point, 2 midpoint, 2 parallel, 1 horizontal, 1 perpendicular, 1 point on line
  measures "d156" diameter of L4 L7
revolve "Вращение6" cut sketch "Эскиз14" angle 360 about axis through (82.45, 0, 0) along (1, 0, 0) contours L2 L3 L1 L4 L0
